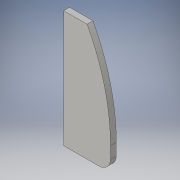
# Autodesk Inventor part: Zachs wing
Saved by Autodesk Inventor 2016 (Build 200138000, 138)
## iProperties
Created: 2018-01-12
Part Number: Zachs wing
Material: Generic
Document SubType Name: Modeling
Designer: fmhs g108
Density: 1 g/cm^3
Appearance: Default
Author: fmhs g108
Autodesk Inventor part; units mm, degrees
ref_plane "YZ Plane" through (0, 0, 0) normal (1, 0, 0) x (0, 1, 0)
ref_plane "XZ Plane" through (0, 0, 0) normal (0, 1, 0) x (-1, 0, 0)
ref_plane "XY Plane" through (0, 0, 0) normal (0, 0, 1) x (1, 0, 0)
sketch "Sketch1" plane through (0, 0, 0) normal (0, 0, 1) x (1, 0, 0)
  line L0 (-10.6635, 0) -> (40.1365, 0)
  line L1 (40.1365, 0) -> (40.1365, 127)
  line L2 (14.7365, 127) -> (-10.6635, 127)
  line L3 (-10.6635, 127) -> (-10.6635, 0)
  line L4 (40.1365, 0) -> (40.1365, 25.4)
  arc A0 (40.1365, 25.4) -> (14.7365, 127) centre (-175.7635, 25.4) ccw
  point P0 (0, 0)
  dimension "d0" = 50.8
  dimension "d1" = 127
  dimension "d2" = 25.4
  constraints: 10 end point, 2 parallel, 2 point on circle, 1 centre point, 1 horizontal, 1 perpendicular, 1 point on line, 1 tangent
  measures "d0" distance of L2.end L1.end
  measures "d1" distance of L1.end L0.end
  measures "d2" distance of L0.end L4.end
extrude "Extrusion1" add sketch "Sketch1" along normal blind 6.35
fillet "Fillet1" radius 12.7 1 edges at (40.1365, 0, 3.175)
body "Solid1"
